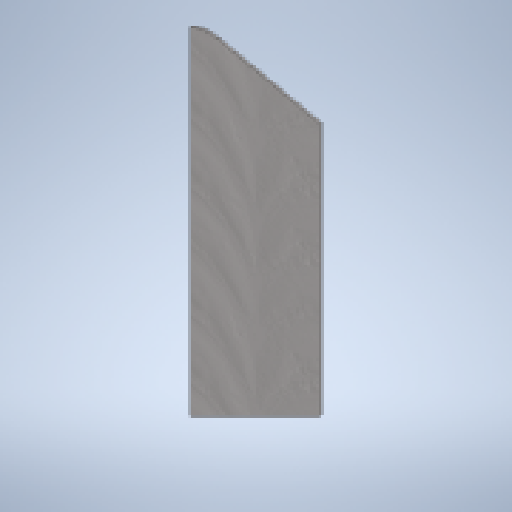
# Autodesk Inventor part: pokrywa prawa
Saved by Autodesk Inventor 2023 (Build 270158000, 158)
## iProperties
Created: 2022-10-11
Part Number: pokrywa prawa
Material: Stal miękka, spawana
Document SubType Name: Modeling
Designer: komputer
Density: 7.85 g/cm^3
Appearance: Spawane — stal miękka
Author: komputer
Autodesk Inventor part; units mm, degrees
ref_plane "YZ Plane" through (0, 0, 0) normal (1, 0, 0) x (0, 1, 0)
ref_plane "XZ Plane" through (0, 0, 0) normal (0, 1, 0) x (-1, 0, 0)
ref_plane "XY Plane" through (0, 0, 0) normal (0, 0, 1) x (1, 0, 0)
sketch "Sketch1" plane through (0, 0, 0) normal (0, 0, 1) x (1, 0, 0)
  line L0 (-17.5, -33.2499) -> (-17.5, 57.9837) projected
  arc A0 (-10.0449, 58.8745) -> (-17.5, 57.9837) centre (-12.5, 47.7794) ccw projected
  line L1 (-10.0449, 58.8745) -> (17.5, 52.7794) projected
  line L2 (17.5, 52.7794) -> (17.5, -15.7501) projected
  line L3 (17.5, -15.7501) -> (-17.5, -33.2499) projected
  line L4 (0.5, 7.1892) -> (0.5, 22.231) projected
  line L5 (0.5, 22.231) -> (-5.8925, 22.231) projected
  line L6 (-5.8925, 22.231) -> (-5.8925, 7.1892) projected
  line L7 (-5.8925, 7.1892) -> (0.5, 7.1892) projected
  point P0 (0, 0)
extrude "Extrusion1" add sketch "Sketch1" along normal blind 0.5 contours L0 A0 L1 L2 L3 | L7 L6 L5 L4
body "Solid1"
